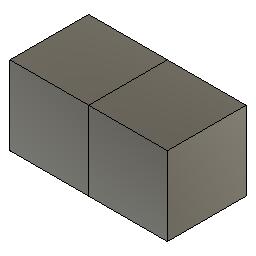
BooleanIntersectContained (Autodesk Fusion 360 design; units mm, degrees)
Autodesk Fusion 360 part; units mm, degrees
sketch "Sketch1" plane through (0, 0, 0) normal (0, 0, 1) x (1, 0, 0)
  line L0 (0, 0) -> (-10, 0)
  line L1 (-10, 0) -> (-10, 10)
  line L2 (-10, 10) -> (0, 10)
  line L3 (0, 10) -> (0, 0)
  line L4 (-8, 8) -> (-3.4733, 8)
  line L5 (-3.4733, 8) -> (-3.4733, 2.3489)
  line L6 (-3.4733, 2.3489) -> (-8, 2.3489)
  line L7 (-8, 2.3489) -> (-8, 8)
  line L8 (-10, 0) -> (10, 0)
  line L9 (10, 0) -> (10, 10)
  line L10 (10, 10) -> (-10, 10)
  line L11 (-10, 10) -> (-10, 0)
  constraint horizontal L0
  constraint vertical L1
  constraint horizontal L2
  constraint vertical L3
  constraint coincident L0.start L3.end
  constraint horizontal L4
  constraint vertical L5
  constraint horizontal L6
  constraint vertical L7
  constraint horizontal L8
  constraint vertical L9
  constraint horizontal L10
  constraint vertical L11
extrude "Extrude1" add sketch "Sketch1" along normal blind 10 contours L0 L1 L2 L3 L8 L10 L11 | L3 L8 L9 L10 | L4 L5 L6 L7 makes body 1
extrude "Extrude1'" add sketch "Sketch1" along normal blind 10 separate body contours L0 L1 L2 L3 L8 L10 L11 | L4 L5 L6 L7 makes body 2 in component "Tool"
extrude "Extrude2" add sketch "Sketch1" along normal blind 5 separate body contours L4 L5 L6 L7 makes body 3 in component "Tool"
component "Tool" placed x (1, 0, 0) y (0, 1, 0) z (0, 0, 1) at (0, 0, 0)
